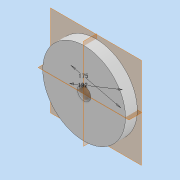
# Autodesk Inventor part: gear2
Saved by Autodesk Inventor 2022 (Build 260153000, 153)
## iProperties
Created: 2023-12-21
Part Number: gear2
Material: 一般
Document SubType Name: Modeling
Designer: ktamu
Density: 1 g/cm^3
Appearance: 既定
Author: ktamu
Autodesk Inventor part; units mm, degrees
sketch "スケッチ1" plane through (0, 0, 0) normal (0, 0, 1) x (1, 0, 0)
  circle A0 centre (0, 0) radius 140
  arc A1 (-6.6994, 21.4795) -> (7, 21.3834) centre (0, 0) ccw
  line L0 (0, 22.5) -> (0, 17)
  line L1 (0, 22.5) -> (0, 26.3)
  line L2 (0, 26.3) -> (7, 26.3)
  line L3 (7, 26.3) -> (7, 21.3834)
  line L4 (7, 17) -> (0, 17)
  line L5 (-6.6994, 21.4795) -> (-6.6994, 26.3)
  line L6 (-6.6994, 26.3) -> (0, 26.3)
  dimension "d0" = 280
  dimension "d1" = 45
  dimension "d2" = 5.5
  dimension "d3" = 3.8
  dimension "d4" = 7
  constraints: 14 end point, 3 perpendicular, 2 centre point, 2 coincident, 2 point on circle, 2 vertical, 1 collinear, 1 horizontal, 1 point on line
  measures "d0" diameter of A0
  measures "d1" diameter of A1
  measures "d2" distance of L0.end L0.start
  measures "d3" distance of L0.start L1.end
  measures "d4" distance of L1.end L2.end
extrude "押し出し1" add sketch "スケッチ1" along normal blind 40
sketch "スケッチ2" plane through (0, 0, 0) normal (0, 0, 1) x (1, 0, 0)
  arc A0 (-6.6994, 21.4795) -> (7, 21.3834) centre (0, 0) ccw projected
  circle A1 centre (0, 0) radius 96 construction
  circle A2 centre (0, 0) radius 87.5 construction
  dimension "d7" = 192
  dimension "d8" = 175
  constraints: 2 centre point, 2 coincident
  measures "d7" diameter of A1
  measures "d8" diameter of A2
